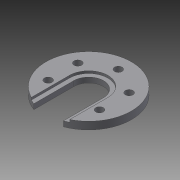
# Autodesk Inventor part: Effector_GrooveMount
Saved by Autodesk Inventor 2014 (Build 180170000, 170)
## iProperties
Created: 2014-01-10
Part Number: Effector_GrooveMount
Material: Generic
Document SubType Name: Modeling
Designer: ThatOtherGuy
Density: 1 g/cm^3
Mass: 2.10677 g
Surface Area: 20.3966 cm^2
Volume: 2.10677 cm^3
Appearance: Default
Author: ThatOtherGuy
Autodesk Inventor part; units mm, degrees
ref_plane "YZ Plane" through (0, 0, 0) normal (1, 0, 0) x (0, 1, 0)
ref_plane "XZ Plane" through (0, 0, 0) normal (0, 1, 0) x (-1, 0, 0)
ref_plane "XY Plane" through (0, 0, 0) normal (0, 0, 1) x (1, 0, 0)
sketch "Sketch1" plane through (0, 0, 0) normal (0, 0, 1) x (1, 0, 0)
  arc A0 (6.25, 0) -> (-6.25, 0) centre (0, 0) ccw
  arc A1 (8.1, 0) -> (-8.1, 0) centre (0, 0) ccw
  arc A2 (8.1, -9.5205) -> (-8.1, -9.5205) centre (0, 0) ccw
  arc A3 (6.25, -16.8801) -> (-6.25, -16.8801) centre (0, 0) ccw
  line L0 (-6.25, 0) -> (-6.25, -16.8801)
  line L1 (6.25, 0) -> (6.25, -16.8801)
  line L2 (8.1, 0) -> (8.1, -16.0745)
  line L3 (-8.1, 0) -> (-8.1, -16.0745)
  circle A4 centre (0, 12.5) radius 1.6
  circle A5 centre (-10.8253, 6.25) radius 1.6
  circle A6 centre (-10.8253, -6.25) radius 1.6
  circle A7 centre (0, -12.5) radius 1.6
  circle A8 centre (10.8253, -6.25) radius 1.6
  circle A9 centre (10.8253, 6.25) radius 1.6
  dimension "d0" = 12.5
  dimension "d2" = 16.2
  dimension "d3" = 25
  dimension "d4" = 36
  dimension "d5" = 3.2
  dimension "d8" = 360
  constraints: 11 point on circle, 10 centre point, 8 end point, 4 coincident, 4 tangent, 3 parallel, 2 point on line, 1 vertical, 13 other
  measures "d0" diameter of A0
  measures "d2" diameter of A1
  measures "d3" diameter of A2
  measures "d4" diameter of A3
  measures "d5" diameter of A4
extrude "Extrusion1" add sketch "Sketch1" along normal blind 2.175 contours A0 L0 A3 L3 A1 L2 L1
extrude "Extrusion2" add sketch "Sketch1" along normal blind 3.175 contours L2 A2 A8 A9 A4 A5 A6 L3 A3 | L2 A1 L3 A2 A6 A5 A4 A9 A8 | A8 A2 | A2 A8 | A6 A2 | A2 A6 | A9 A2 | A2 A9 | A5 A2 | A2 A5 | A4 A2 | A2 A4
extrude "Extrusion3" cut sketch "Sketch1" along normal through all contours A8 A2 | A2 A8 | A6 A2 | A2 A6 | A9 A2 | A2 A9 | A5 A2 | A2 A5 | A4 A2 | A2 A4
equation "\"d12\" = THICKA"
equation "\"THICKA\" = 3.175"
equation "\"THICKB\" = 6.731"
equation "\"THICKC\" = 12.7"
equation "\"BALLDIA\" = 12"
equation "\"MAGDIA\" = 9.5"
equation "\"THICKPLY\" = 5"
body "Solid1"
